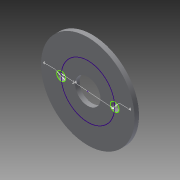
# Autodesk Inventor part: AlatetMotor
Saved by Autodesk Inventor 2015 SP1 (Build 190203100, 203)
## iProperties
Created: 2014-09-27
Part Number: AlatetMotor
Material: Generic
Document SubType Name: Modeling
Designer: laca
Density: 1 g/cm^3
Appearance: Default
Mass: 2.51715 g
Surface Area: 29.0282 cm^2
Volume: 2.51715 cm^3
Author: laca
Autodesk Inventor part; units mm, degrees
ref_plane "YZ Plane" through (0, 0, 0) normal (1, 0, 0) x (0, 1, 0)
ref_plane "XZ Plane" through (0, 0, 0) normal (0, 1, 0) x (-1, 0, 0)
ref_plane "XY Plane" through (0, 0, 0) normal (0, 0, 1) x (1, 0, 0)
sketch "Sketch1" plane through (0, 0, 0) normal (0, 0, 1) x (1, 0, 0)
  circle A0 centre (0, 0) radius 5.6906
  circle A1 centre (0, 0) radius 21
  dimension "d0" = 42
  constraints: 2 centre point, 2 coincident
  measures "d0" diameter of A1
extrude "Extrusion1" add sketch "Sketch1" along normal blind 2
sketch "Sketch2" plane through (0, 0, 2) normal (0, 0, 1) x (1, 0, 0)
  circle A0 centre (0, 0) radius 12
  circle A1 centre (-12, 0) radius 2
  circle A2 centre (12, 0) radius 2
  dimension "d3" = 24
  dimension "d4" = 4
  dimension "d5" = 4
  constraints: 3 centre point, 2 point on circle, 1 coincident
  measures "d3" diameter of A0
  measures "d4" diameter of A1
  measures "d5" diameter of A2
extrude "Extrusion2" cut sketch "Sketch2" against normal through all contours A0 A2 | A0 A2 | A1 A0 | A0 A1
sketch "Sketch3" plane through (0, 0, 2) normal (0, 0, 1) x (1, 0, 0)
  point P0 (0, 12)
  point P1 (0, -12)
hole "Hole1" at (0, 12, 2) at (0, -12, 2) direction (0, 0, -1) diameter 3.4 depth 2
body "Solid1"
